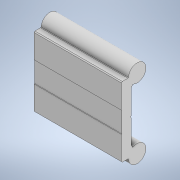
# Autodesk Inventor part: WS_10_40_custom_length
Saved by Autodesk Inventor 2020 (Build 240168000, 168)
## iProperties
Created: 2022-03-14
Part Number: WS_10_40_custom_length
Material: Ogólny
Document SubType Name: Modeling
Designer: mikoma
Density: 1 g/cm^3
Appearance: Domyślna
Author: mikoma
Autodesk Inventor part; units mm, degrees
ref_plane "YZ Plane" through (0, 0, 0) normal (1, 0, 0) x (0, 1, 0)
ref_plane "XZ Plane" through (0, 0, 0) normal (0, 1, 0) x (-1, 0, 0)
ref_plane "XY Plane" through (0, 0, 0) normal (0, 0, 1) x (1, 0, 0)
sketch "Szkic1" plane through (0, 0, 0) normal (1, 0, 0) x (0, 1, 0)
  line L0 (13.7, -0.2) -> (25.3, -0.2)
  line L1 (13.5, 0) -> (13.7, -0.2)
  line L2 (0, 0) -> (13.5, 0)
  line L3 (-0.5, -0.5) -> (0, 0)
  line L4 (-0.5, -3.7085) -> (-0.5, -0.5)
  arc A0 (-0.783, -4.008) -> (-0.5, -3.7085) centre (-0.8, -3.7085) ccw
  arc A1 (-0.783, -4.008) -> (3.9514, -6.7229) centre (-0.5, -9) ccw
  arc A2 (4.0685, -6.3265) -> (3.9514, -6.7229) centre (4.2185, -6.5863) ccw
  line L5 (5.5, -5.5) -> (4.0685, -6.3265)
  line L6 (19, -5.5) -> (5.5, -5.5)
  line L7 (19.5, -5.2113) -> (19, -5.5)
  line L8 (20, -5.5) -> (19.5, -5.2113)
  line L9 (33.5, -5.5) -> (20, -5.5)
  line L10 (34.9315, -6.3265) -> (33.5, -5.5)
  arc A3 (35.0486, -6.7229) -> (34.9315, -6.3265) centre (34.7815, -6.5863) ccw
  arc A4 (35.0486, -6.7229) -> (39.783, -4.008) centre (39.5, -9) ccw
  arc A5 (39.5, -3.7085) -> (39.783, -4.008) centre (39.8, -3.7085) ccw
  line L11 (39.5, -0.5) -> (39.5, -3.7085)
  line L12 (39, 0) -> (39.5, -0.5)
  line L13 (25.5, 0) -> (39, 0)
  line L14 (25.3, -0.2) -> (25.5, 0)
  point P0 (19.5, 0)
  constraints: 30 end point, 12 point on circle, 8 tangent, 7 parallel, 6 centre point, 5 horizontal, 4 equal radius, 3 vertical, 1 perpendicular, 43 other
extrude "Wyciągnięcie proste1" add sketch "Szkic1" along normal blind 50
